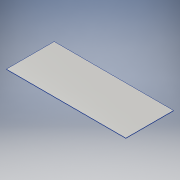
# Autodesk Inventor part: ballRamp
Saved by Autodesk Inventor 2016 SP1 (Build 200210100, 210)
## iProperties
Created: 2016-01-19
Part Number: ballRamp
Material: Aluminum 6061
Document SubType Name: Modeling
Designer: steele
Density: 2.7 g/cm^3
Appearance: Aluminum - Flat
Author: steele
Autodesk Inventor part; units mm, degrees
ref_plane "YZ Plane" through (0, 0, 0) normal (1, 0, 0) x (0, 1, 0)
ref_plane "XZ Plane" through (0, 0, 0) normal (0, 1, 0) x (-1, 0, 0)
ref_plane "XY Plane" through (0, 0, 0) normal (0, 0, 1) x (1, 0, 0)
sketch "Sketch1" plane through (0, 0, 0) normal (0, 1, 0) x (-1, 0, 0)
  line L0 (254, 101.6) -> (-254, 101.6)
  line L1 (-254, 101.6) -> (-254, -101.6)
  line L2 (-254, -101.6) -> (254, -101.6)
  line L3 (254, -101.6) -> (254, 101.6)
  line L4 (254, 101.6) -> (-254, -101.6) construction
  line L5 (-254, 101.6) -> (254, -101.6) construction
  point P0 (0, 0)
  dimension "d0" = 203.2
  dimension "d1" = 508
  constraints: 12 end point, 2 midpoint, 2 parallel, 1 horizontal, 1 perpendicular
  measures "d0" distance of L2.end L0.start
  measures "d1" distance of L0.start L0.end
extrude "Extrusion1" add sketch "Sketch1" along normal blind 1.5875
equation "\"d0\" = ballRampWidth"
equation "\"d1\" = ballRampLength"
equation "\"d2\" = ballRampThickness"
equation "\"ballRampWidth\" = 203.2"
equation "\"ballRampLength\" = 508"
equation "\"ballRampThickness\" = 1.5875"
body "Solid1"
